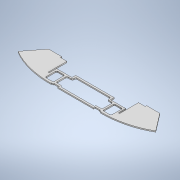
# Autodesk Inventor part: bulkhead_main
Saved by Autodesk Inventor 2020.3 (Build 243373010, 373A)
## iProperties
Created: 2020-05-22
Part Number: bulkhead_main
Material: Generic
Document SubType Name: Modeling
Designer: kardo
Density: 1 g/cm^3
Appearance: Default
Mass: 10.1911 g
Surface Area: 121.313 cm^2
Volume: 10.1911 cm^3
Author: kardo
Autodesk Inventor part; units mm, degrees
ref_plane "YZ Plane" through (0, 0, 0) normal (1, 0, 0) x (0, 1, 0)
ref_plane "XZ Plane" through (0, 0, 0) normal (0, 1, 0) x (-1, 0, 0)
ref_plane "XY Plane" through (0, 0, 0) normal (0, 0, 1) x (1, 0, 0)
derived "base_sketch.ipt"
sketch "stringer" plane through (0, 0, 0) normal (1, 0, 0) x (0, 1, 0)
  line L0 (-306, 11.475) -> (0, 0)
  line L1 (-306, 31.875) -> (-306, 11.475)
  line L2 (-412.4622, 0) -> (310.4457, 0)
  line L3 (0, -13.6228) -> (0, 64.3297)
  line L4 (0, 0) -> (122.4, 8.559)
  line L5 (-306, 31.875) -> (-153, 45.9) construction
  line L6 (-153, 45.9) -> (0, 45.9) construction
  line L7 (0, 45.9) -> (102, 45.9) construction
  line L8 (102, 45.9) -> (204, 35.7) construction
  line L9 (122.4, 8.559) -> (204, 14.2651) construction
  spline S0 degree 4 poles (-306, 31.875) (-229.6805, 38.871) (-153.0004, 41.6957) (-76.5755, 45.9) (0, 45.9) knots 0 0 0 0 0 1 1 1 1 1
  spline S1 degree 4 poles (0, 45.9) (51.0599, 45.9) (102.0004, 42.8427) (153.143, 40.7857) (204, 35.7) knots 0 0 0 0 0 1 1 1 1 1
  spline S2 degree 4 poles (122.4, 8.559) (129.6243, 9.0642) (155.3021, 10.8598) (183.5774, 20.1745) (192.0601, 27.4338) (204, 35.7) knots 0 0 0 0 0 0.281346 1 1 1 1 1
  point P0 (-153, 41.6925)
  point P1 (102, 42.84)
  point P2 (163.2, 15.056)
  point P3 (187.68, 24.9131)
sketch "bulkhead_main" plane through (0, 0, 0) normal (0, 1, 0) x (-1, 0, 0)
  line L0 (0, 19.935) -> (28.764, 19.935)
  line L1 (28.764, 19.935) -> (28.764, 13.529)
  line L2 (28.764, 13.529) -> (62.322, 13.529)
  line L3 (0, 0) -> (-11.5056, 0)
  line L4 (-11.5056, 0) -> (-11.5056, -2.4868)
  line L5 (-11.5056, -2.4868) -> (-34.5168, -2.4868)
  line L6 (-34.5168, -2.4868) -> (-57.528, 27.54)
  line L7 (19.176, 46.818) -> (62.322, 46.818)
  line L8 (0, 19.935) -> (0, 0)
  line L9 (86.7165, 0) -> (-84.045, 0)
  line L10 (0, -13.6228) -> (0, 64.3297)
  line L11 (62.322, 46.818) -> (62.322, 13.529)
  spline S0 degree 4 poles (-57.528, 27.54) (-46.0483, 34.2051) (-30.6129, 40.5281) (-11.2214, 45.0414) (8.3201, 46.818) (15.5662, 46.818) (19.176, 46.818) knots 0 0 0 0 0 0.630279 0.815816 1 1 1 1 1
  line L12 (0, 35.7) -> (-57.528, 27.54) construction
  line L13 (-11.5056, -2.4868) -> (0, -2.4868) construction
  line L14 (0, -2.4868) -> (0, 0) construction
  point P0 (0, 45.9)
  point P1 (-38.352, 36.72)
  point P2 (-19.176, 42.5952)
  point P3 (0, 13.529)
ref_plane "bulkhead_main_plane" through (0, 0, 0) normal (0, 1, 0) x (-1, 0, 0)
sketch "Sketch3" plane through (0, 0, 0) normal (0, 1, 0) x (-1, 0, 0)
  spline S0 degree 4 poles (-57.528, 27.54) (-46.0483, 34.2051) (-30.6129, 40.5281) (-11.2214, 45.0414) (8.3201, 46.818) (15.5662, 46.818) (19.176, 46.818) knots 0 0 0 0 0 0.630279 0.815816 1 1 1 1 1 projected
  line L0 (19.176, 46.818) -> (62.322, 46.818) projected
  line L1 (62.322, 46.818) -> (62.322, 13.529) projected
  line L2 (28.764, 13.529) -> (62.322, 13.529) projected
  line L3 (28.764, 19.935) -> (28.764, 13.529) projected
  line L4 (0, 19.935) -> (28.764, 19.935) projected
  line L5 (0, 19.935) -> (0, 0) projected
  line L6 (0, 0) -> (-11.5056, 0) projected
  line L7 (-11.5056, -2.4868) -> (-34.5168, -2.4868) projected
  line L8 (-11.5056, 0) -> (-11.5056, -2.4868) projected
  line L9 (-34.5168, -2.4868) -> (-57.528, 27.54) projected
  line L10 (0, 32.9175) -> (2, 32.9175)
  line L11 (2, 32.9175) -> (2, 19.935)
  line L12 (0, 32.9175) -> (0, 19.935)
  line L13 (0, 32.9175) -> (0, 45.9) construction
  line L14 (2, 32.9175) -> (2, 46.1141) construction
  line L15 (7, 43.1141) -> (17.176, 43.1141)
  line L16 (19.176, 41.1141) -> (19.176, 24.935)
  line L17 (17.176, 22.935) -> (7, 22.935)
  line L18 (5, 24.935) -> (5, 41.1141)
  arc A0 (7, 43.1141) -> (5, 41.1141) centre (7, 41.1141) ccw
  arc A1 (19.176, 41.1141) -> (17.176, 43.1141) centre (17.176, 41.1141) ccw
  arc A2 (17.176, 22.935) -> (19.176, 24.935) centre (17.176, 24.935) ccw
  arc A3 (5, 24.935) -> (7, 22.935) centre (7, 24.935) ccw
  line L19 (24.176, 41.418) -> (31.176, 41.418)
  line L20 (62.322, 16.529) -> (33.764, 16.529)
  line L21 (31.764, 18.529) -> (31.764, 19.935)
  line L22 (22.176, 24.935) -> (22.176, 39.418)
  arc A4 (24.176, 41.418) -> (22.176, 39.418) centre (24.176, 39.418) ccw
  arc A5 (31.764, 18.529) -> (33.764, 16.529) centre (33.764, 18.529) ccw
  line L23 (24.4815, 22.535) -> (29.4585, 22.335)
  spline S1 degree 3 poles (22.176, 24.935) (22.176, 23.671) (23.2185, 22.5858) (24.4815, 22.535) knots 0 0 0 0 1 1 1 1
  spline S2 degree 3 poles (29.4585, 22.335) (30.7215, 22.2843) (31.764, 21.199) (31.764, 19.935) knots 0 0 0 0 1 1 1 1
  line L24 (22.176, 24.935) -> (24.4815, 22.535) construction
  line L25 (29.4585, 22.335) -> (31.764, 19.935) construction
  line L26 (22.176, 24.935) -> (31.764, 19.935) construction
  line L27 (29.4585, 22.335) -> (31.764, 22.2424) construction
  line L28 (31.764, 22.2424) -> (31.764, 19.935) construction
  line L29 (19.176, 46.818) -> (19.176, 45.618)
  line L30 (19.176, 45.618) -> (22.176, 45.618)
  line L31 (22.176, 45.618) -> (22.176, 44.418)
  line L32 (22.176, 44.418) -> (31.176, 44.418)
  line L33 (31.176, 44.418) -> (31.176, 46.818)
  line L34 (22.176, 45.618) -> (25.176, 45.618) construction
  line L35 (25.176, 45.618) -> (25.176, 46.818) construction
  line L36 (34.0605, 43.818) -> (62.322, 43.818)
  spline S3 degree 3 poles (31.176, 41.418) (31.7112, 41.418) (32.2056, 41.733) (32.4317, 42.218) knots 0 0 0 0 1 1 1 1
  spline S4 degree 3 poles (34.0605, 43.818) (33.5254, 43.818) (33.031, 43.503) (32.8048, 43.018) knots 0 0 0 0 1 1 1 1
  line L37 (32.8048, 43.018) -> (32.4317, 42.218)
  line L38 (31.176, 41.418) -> (32.0587, 41.418) construction
  line L39 (32.0587, 41.418) -> (32.4317, 42.218) construction
  line L40 (32.8048, 43.018) -> (33.1778, 43.818) construction
  line L41 (33.1778, 43.818) -> (34.0605, 43.818) construction
  line L42 (31.176, 41.418) -> (34.0605, 43.818) construction
  point P0 (26.97, 22.435)
  point P1 (32.6183, 42.618)
  dimension "d1" = 2
  dimension "d4" = 3
  dimension "d6" = 3
  dimension "d7" = 3
  dimension "d8" = 2
  dimension "d12" = 3
  dimension "d13" = 3
  dimension "d14" = 2
  dimension "d24" = 5
  dimension "d27" = 0.2
  dimension "d28" = 2
  dimension "d29" = 3
  dimension "d33" = 1.2
  dimension "d34" = 1.2
  dimension "d35" = 6
  dimension "d36" = 6
  dimension "d37" = 3
  dimension "d38" = 3
  dimension "d39" = 115
  constraints: 66 end point, 12 point on circle, 12 tangent, 8 parallel, 8 point on line, 7 collinear, 7 equal length, 6 centre point, 6 perpendicular, 5 vertical, 4 horizontal, 4 midpoint, 3 equal radius, 14 other
  measures "d1" distance of L10.start L10.end
  measures "d4" distance between parallel lines of L18 L11
  measures "d6" distance from line of L14.end L15
  measures "d7" distance between parallel lines of L4 L17
  measures "d8" radius of A0
  measures "d12" distance between parallel lines of L21 L3
  measures "d13" distance between parallel lines of L2 L20
  measures "d14" radius of A4
  measures "d24" distance from line of L22.start L4
  measures "d27" vertical distance of L23.start L23.end
  measures "d28" radius of A5
  measures "d29" distance between parallel lines of L22 L16
  measures "d33" distance of L0.start L29.end
  measures "d34" distance of L30.end L31.end
  measures "d35" distance between parallel lines of L33 L35
  measures "d36" distance between parallel lines of L35 L29
  measures "d37" distance between parallel lines of L19 L32
  measures "d38" distance between parallel lines of L0 L36
  measures "d39" angle of L37 L19
extrude "Extrusion1" add sketch "Sketch3" along normal blind 2 contours S0 L29 L30 L31 L32 L33 L0 L1 L36 S4 L37 S3 L19 A4 L22 S1 L23 S2 L21 A5 L20 L2 L3 L4 L11 L10 L12 L5 L6 L8 L7 L9
mirror "Mirror1" about plane through (-62.322, 0, 13.529) normal (-1, 0, 0) of "Extrusion1"
equation "\"d1\" = stringer_thickness"
equation "\"d2\" = bulkhead_thickness"
equation "\"stringer_thickness\" = 2"
equation "\"bulkhead_thickness\" = 2"
body "Solid1"
